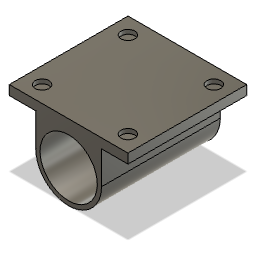
IMU_Tube_Mount_01 v1 (Autodesk Fusion 360 design; units mm, degrees)
Autodesk Fusion 360 part; units mm, degrees
sketch "Sketch1" plane through (0, 0, 0) normal (0, 1, 0) x (1, 0, 0)
  line L0 (14, -14) -> (-14, -14)
  line L1 (-14, -14) -> (-14, 14)
  line L2 (-14, 14) -> (14, 14)
  line L3 (14, 14) -> (14, -14)
  line L4 (14, -14) -> (-14, 14) construction
  line L5 (-14, -14) -> (14, 14) construction
  dimension "d1" = 28
  dimension "d2" = 28
  constraint horizontal L0
  constraint perpendicular L0 L1
  constraint parallel L0 L2
  constraint parallel L1 L3
  constraint coincident L4 origin
  constraint coincident L5 origin
  measures "d1" distance of L1.end L2.end
  measures "d2" distance of L0.end L1.end
extrude "Extrude1" add sketch "Sketch1" along normal blind 18
sketch "Sketch2" plane through (0, 0, 14) normal (0, 0, 1) x (1, 0, 0)
  line L0 (-14, 0) -> (14, 0)
  line L1 (14, 0) -> (14, 18)
  line L2 (14, 18) -> (-14, 18)
  line L3 (-14, 18) -> (-14, 0)
  line L4 (0, 18) -> (0, 0) construction
  circle A0 centre (0, 9) radius 6.75
  circle A1 centre (0, 9) radius 7.75
  line L5 (0, 9) -> (-7.75, 9)
  line L6 (0, 9) -> (7.75, 9)
  line L7 (0, 16.75) -> (-14, 16.75)
  line L8 (0, 16.75) -> (14, 16.75)
  line L9 (-14, 16.75) -> (-6.5677, 4.8857) construction
  line L10 (14, 16.75) -> (6.5677, 4.8857) construction
  point P0 (0, 2.25)
  dimension "d5" = 13.5
  dimension "d18" = 15.5
  dimension "d23" = 14
  constraint midpoint L2 L4.start
  constraint coincident L4.end origin
  constraint midpoint L4 A0.centre
  constraint coincident L4 P0
  constraint coincident A0 P0
  constraint concentric A0 A1
  constraint coincident A0.centre A1.centre
  constraint coincident A1 L5.end
  constraint perpendicular L4 L5
  constraint coincident A1 L6.end
  constraint parallel L5 L6
  constraint horizontal L7
  constraint coincident A1 L7.start
  constraint coincident L4 L7.start
  constraint horizontal L8
  constraint coincident L1 L8.end
  constraint coincident A1 L9.end
  constraint tangent A1 L9
  constraint coincident A1 L10.end
  constraint tangent A1 L10
  measures "d5" diameter of A0
  measures "d18" diameter of A1
  measures "d23" distance of L7.end L9.end
sketch "Sketch3" plane through (0, 18, 0) normal (0, 1, 0) x (-1, 0, 0)
  line L0 (-14, -14) -> (14, -14)
  line L1 (14, -14) -> (14, 14)
  line L2 (14, 14) -> (-14, 14)
  line L3 (-14, 14) -> (-14, -14)
  line L4 (-13, 13) -> (13, 13)
  line L5 (13, 13) -> (13, -13)
  line L6 (13, -13) -> (-13, -13)
  line L7 (-13, -13) -> (-13, 13)
  line L8 (-13, 13) -> (13, -13) construction
  line L9 (13, 13) -> (-13, -13) construction
  line L10 (10.125, -14) -> (10.125, 14) construction
  line L11 (-10.125, -14) -> (-10.125, 14) construction
  line L12 (14, -10.125) -> (-14, -10.125) construction
  line L13 (14, 10.125) -> (-14, 10.125) construction
  circle A0 centre (10.125, 10.125) radius 1.625
  circle A1 centre (10.125, -10.125) radius 1.625
  circle A2 centre (-10.125, -10.125) radius 1.625
  circle A3 centre (-10.125, 10.125) radius 1.625
  dimension "d6" = 26
  dimension "d7" = 26
  dimension "d10" = 2.875
  dimension "d11" = 2.875
  dimension "d12" = 2.875
  dimension "d13" = 2.875
  dimension "d14" = 3.25
  dimension "d15" = 3.25
  dimension "d16" = 3.25
  dimension "d17" = 3.25
  constraint horizontal L4
  constraint perpendicular L4 L5
  constraint parallel L4 L6
  constraint parallel L5 L7
  constraint coincident L8 origin
  constraint coincident L9 origin
  constraint coincident L0 L10.start
  constraint perpendicular L0 L10
  constraint coincident L2 L10.end
  constraint coincident L0 L11.start
  constraint perpendicular L0 L11
  constraint coincident L2 L11.end
  constraint coincident L1 L12.start
  constraint perpendicular L1 L12
  constraint coincident L3 L12.end
  constraint coincident L1 L13.start
  constraint perpendicular L1 L13
  constraint coincident L3 L13.end
  constraint coincident L10 A0.centre
  constraint coincident L13 A0.centre
  constraint coincident L8 A1.centre
  constraint coincident L10 A1.centre
  constraint coincident L12 A2.centre
  constraint coincident L9 A2.centre
  constraint coincident L13 A3.centre
  constraint coincident L11 A3.centre
  measures "d6" distance of L5.end L6.end
  measures "d7" distance of L4.end L5.end
  measures "d10" distance of L5 L10
  measures "d11" distance of L7 L11
  measures "d12" distance of L6 L12
  measures "d13" distance of L4 L13
  measures "d14" diameter of A0
  measures "d15" diameter of A1
  measures "d16" diameter of A2
  measures "d17" diameter of A3
extrude "Extrude2" cut sketch "Sketch2" against normal blind 28 contours A0 L5 L6 | A0 L5 L6
extrude "Extrude3" add sketch "Sketch3" along normal blind 1 contours L0 L1 L2 L3 | L4 L5 L6 L7
sketch "Sketch4" plane through (0, 0, 14) normal (0, 0, 1) x (1, 0, 0)
  line L0 (-14, 16.75) -> (-6.5677, 4.8857)
  line L1 (14, 16.75) -> (6.5677, 4.8857)
  circle A0 centre (0, 9) radius 7.75
  circle A1 centre (0, 9) radius 6.75
  line L2 (0, 9) -> (7.75, 9)
  line L3 (0, 9) -> (-7.75, 9)
  line L4 (0, 18) -> (0, 0)
  line L5 (0, 16.75) -> (-14, 16.75)
  line L6 (13, 18) -> (-13, 18)
  line L7 (-8.5, 18) -> (-11.75, 18)
  line L8 (11.75, 18) -> (8.5, 18)
  line L9 (-8.5, 18) -> (-11.75, 18)
  line L10 (11.75, 18) -> (8.5, 18)
  line L11 (-8.5, 18) -> (-8.5, 0) construction
  line L12 (8.5, 18) -> (8.5, 0) construction
  line L13 (0, 16.75) -> (14, 16.75)
  line L14 (-7.75, 9) -> (-7.75, 18.001)
  line L15 (7.75, 9) -> (7.75, 18.0312)
  line L16 (-14, 16.75) -> (-7.75, 16.75)
  line L17 (14, 16.75) -> (7.75, 16.75)
  line L18 (14, 16.75) -> (14, 0)
  line L19 (14, 0) -> (-14, 0)
  line L20 (-14, 0) -> (-14, 16.75)
  point P0 (0, 9)
  constraint coincident L7.start L9.start
  constraint perpendicular L9 L11
  constraint coincident L8.end L10.end
  constraint perpendicular L8 L12
  constraint vertical L14
  constraint coincident L3.end L14.start
  constraint vertical L15
  constraint coincident L2.end L15.start
  constraint coincident L0.start L5.end
  constraint coincident L14 L16.end
  constraint coincident L5 L16.end
  constraint coincident L1.start L13.end
  constraint coincident L13 L17.end
  constraint coincident L15 L17.end
  constraint perpendicular L13 L18
  constraint perpendicular L11 L19
extrude "Extrude4" cut sketch "Sketch4" against normal blind 28 contours L0 A0 L5 L14 L16 | L0 A0 L4 L19 L20 | L1 A0 L4 L18 L19 | L1 A0 L13 L15 L17
